Autodesk Inventor part; units mm, degrees
(part 2 of 2)
  arc A214 (18.0089, 12.613) -> (14.659, 12.9654) centre (16.2027, 11.5417) ccw projected
  arc A215 (17.3596, -8.3042) -> (18.0089, 12.613) centre (1.2373, 2.6649) ccw projected
  arc A216 (13.9943, -8.4482) -> (17.3596, -8.3042) centre (15.6233, -7.1229) ccw projected
  line L59 (13.9943, -8.4482) -> (7.5036, -0.4695) projected
  arc A217 (7.0857, 1.3248) -> (7.5036, -0.4695) centre (9.1327, 0.8557) ccw projected
  line L60 (-9.8758, -10.0921) -> (-1.8971, -3.6014) projected
  arc A218 (-0.1028, -3.1835) -> (-1.8971, -3.6014) centre (-0.5719, -5.2305) ccw projected
  arc A219 (-0.1028, -3.1835) -> (2.2121, -3.2554) centre (1.2373, 2.6649) ccw projected
  arc A220 (3.977, -3.7838) -> (2.2121, -3.2554) centre (2.5533, -5.3275) ccw projected
  line L61 (3.977, -3.7838) -> (11.5378, -10.7568) projected
  arc A221 (11.1854, -14.1066) -> (11.5378, -10.7568) centre (10.1141, -12.3005) ccw projected
  arc A222 (-9.7318, -13.4574) -> (11.1854, -14.1066) centre (1.2373, 2.6649) ccw projected
  arc A223 (-9.8758, -10.0921) -> (-9.7318, -13.4574) centre (-8.5506, -11.7211) ccw projected
  line L62 (-11.5197, 13.778) -> (-5.029, 5.7993) projected
  arc A224 (-4.6111, 4.005) -> (-5.029, 5.7993) centre (-6.6581, 4.4741) ccw projected
  arc A225 (-4.6111, 4.005) -> (-4.683, 1.6901) centre (1.2373, 2.6649) ccw projected
  arc A226 (-5.2114, -0.0748) -> (-4.683, 1.6901) centre (-6.7551, 1.3489) ccw projected
  line L63 (-5.2114, -0.0748) -> (-12.1844, -7.6356) projected
  arc A227 (-15.5343, -7.2832) -> (-12.1844, -7.6356) centre (-13.7281, -6.2119) ccw projected
  arc A228 (-14.885, 13.6341) -> (-15.5343, -7.2832) centre (1.2373, 2.6649) ccw projected
  arc A229 (-11.5197, 13.778) -> (-14.885, 13.6341) centre (-13.1487, 12.4528) ccw projected
  circle A230 centre (1.2373, 2.6649) radius 8.025
  point P0 (0, 0)
  point P1 (-5.9594, -0.8859)
  point P2 (-2.753, -4.2977)
  point P3 (4.7881, -4.5318)
  point P4 (8.1999, -1.3254)
  point P5 (8.434, 6.2157)
  point P6 (5.2276, 9.6275)
  point P7 (-2.3135, 9.8616)
  point P8 (-5.7253, 6.6552)
  dimension "d20" = 16.05
  constraints: 1 centre point, 1 coincident
  measures "d20" diameter of A230
extrude "押し出し2" cut sketch "スケッチ3" against normal blind 1 contours A205 A204 A203 L51 A230 L58 A213 A212 A217 L59 L61 A220 A219 A218 L60 L63 A226 A225 A224 L62 L50
